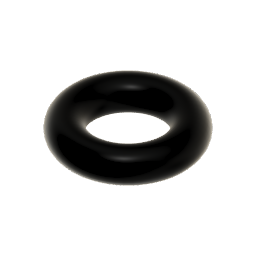
Rubber_6mm (Autodesk Fusion 360 design; units mm, degrees)
Autodesk Fusion 360 part; units mm, degrees
sketch "Sketch1" plane through (0, 0, 0) normal (0, 0, 1) x (1, 0, 0)
  circle A0 centre (0, 0) radius 3
  circle A1 centre (0, 0) radius 1.5
  dimension "d1" = 6
  dimension "d2" = 3
  constraint coincident A0.centre A1.centre
  measures "d1" diameter of A0
  measures "d2" diameter of A1
extrude "Extrude1" add sketch "Sketch1" along normal blind 1.5
fillet "Fillet1" radius 0.75 4 edges at (-2.797, -1.0848, 1.5) (-2.797, -1.0848, 0) (-1.3985, 0.5424, 1.5) (-1.3985, 0.5424, 0)
equation "d1 = outerDiameter"
equation "d2 = innerDiameter"
equation "d3 = height"
equation "d6 = height / 2"
equation "outerDiameter = 6 mm"
equation "innerDiameter = 3 mm"
equation "height = 1.5 mm"
named bodies: "Rubber_6mm"
